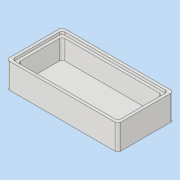
# Autodesk Inventor part: BackupNanoCasePart1
Saved by Autodesk Inventor 2017 (Build 210142000, 142)
## iProperties
Created: 2018-02-21
Part Number: BackupNanoCasePart1
Material: ABS Plastic
Document SubType Name: Modeling
Designer: Derek Wider
Density: 1.06 g/cm^3
Appearance: Smooth - White
Author: Derek Wider
Autodesk Inventor part; units mm, degrees
ref_plane "YZ Plane" through (0, 0, 0) normal (1, 0, 0) x (0, 1, 0)
ref_plane "XZ Plane" through (0, 0, 0) normal (0, 1, 0) x (-1, 0, 0)
ref_plane "XY Plane" through (0, 0, 0) normal (0, 0, 1) x (1, 0, 0)
sketch "Sketch1" plane through (0, 0, 0) normal (0, 1, 0) x (-1, 0, 0)
  line L0 (0, 0) -> (50.8, 0)
  line L1 (50.8, 0) -> (50.8, -25.4)
  line L2 (50.8, -25.4) -> (0, -25.4)
  line L3 (0, -25.4) -> (0, 0)
  line L4 (48.26, -22.86) -> (48.26, -2.54)
  line L5 (48.26, -2.54) -> (2.54, -2.54)
  line L6 (2.54, -2.54) -> (2.54, -22.86)
  line L7 (2.54, -22.86) -> (48.26, -22.86)
  dimension "d0" = 50.8
  dimension "d1" = 25.4
  dimension "d2" = 2.54
  constraints: 16 end point, 4 parallel, 2 perpendicular, 1 horizontal, 3 other
  measures "d0" distance of L1.end L2.end
  measures "d1" distance of L0.end L1.end
  measures "d2" distance between parallel lines of L1 L4
extrude "Extrusion1" add sketch "Sketch1" along normal blind 11.43
extrude "Extrusion2" add sketch "Sketch1" along normal blind 1.27 contours L7 L6 L5 L4
sketch "Sketch2" plane through (0, 11.43, 0) normal (0, 1, 0) x (1, 0, 0)
  line L0 (-48.26, 22.86) -> (-2.54, 22.86) projected
  line L1 (-2.54, 22.86) -> (-2.54, 2.54) projected
  line L2 (-2.54, 2.54) -> (-48.26, 2.54) projected
  line L3 (-48.26, 2.54) -> (-48.26, 22.86) projected
  line L4 (-50.8, 0) -> (0, 0) projected
  line L5 (0, 0) -> (0, 25.4) projected
  line L6 (0, 25.4) -> (-50.8, 25.4) projected
  line L7 (-50.8, 25.4) -> (-50.8, 0) projected
  line L8 (-49.53, 24.13) -> (-1.27, 24.13)
  line L9 (-1.27, 24.13) -> (-1.27, 1.27)
  line L10 (-1.27, 1.27) -> (-49.53, 1.27)
  line L11 (-49.53, 1.27) -> (-49.53, 24.13)
  dimension "d7" = 1.27
  constraints: 8 end point, 3 other
  measures "d7" distance between parallel lines of L3 L11
extrude "Extrusion3" cut sketch "Sketch2" against normal blind 1.27 contours L8 L9 L10 L11
fillet "Fillet1" radius 1.27 12 edges at (-2.54, 5.715, -2.54) (-1.27, 10.795, -1.27) (0, 5.715, 0) (-50.8, 5.715, 0) (-49.53, 10.795, -1.27) (-48.26, 5.715, -2.54) (-50.8, 5.715, -25.4) (-49.53, 10.795, -24.13) (-48.26, 5.715, -22.86) (0, 5.715, -25.4) (-1.27, 10.795, -24.13) (-2.54, 5.715, -22.86)
body "Solid1"
